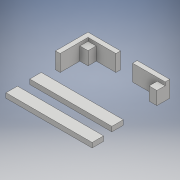
# Autodesk Inventor part: Suporte_proto
Saved by Autodesk Inventor 2018 (Build 220112000, 112)
## iProperties
Created: 2018-05-07
Part Number: Suporte_proto
Material: Genérico
Document SubType Name: Modeling
Designer: mirre
Density: 1 g/cm^3
Appearance: Padrão
Author: mirre
Autodesk Inventor part; units mm, degrees
ref_plane "YZ Plane" through (0, 0, 0) normal (1, 0, 0) x (0, 1, 0)
ref_plane "XZ Plane" through (0, 0, 0) normal (0, 1, 0) x (-1, 0, 0)
ref_plane "XY Plane" through (0, 0, 0) normal (0, 0, 1) x (1, 0, 0)
sketch "Esboço1" plane through (0, 0, 0) normal (0, 0, 1) x (1, 0, 0)
  line L0 (0, 20) -> (0, 0)
  line L1 (45, 0) -> (45, 5)
  line L2 (45, 5) -> (50, 5)
  line L3 (50, 5) -> (50, 0)
  line L4 (50, 0) -> (45, 0)
  line L5 (0, 30) -> (0, 50)
  line L6 (8, 47) -> (8, 42)
  line L7 (8, 42) -> (3, 42)
  line L8 (3, 42) -> (3, 30)
  line L9 (3, 30) -> (0, 30)
  line L10 (30, 50) -> (50, 50)
  line L11 (50, 50) -> (50, 42)
  line L12 (50, 42) -> (45, 42)
  line L13 (45, 42) -> (45, 47)
  line L14 (45, 47) -> (30, 47)
  line L15 (30, 47) -> (30, 50)
  line L16 (0, 50) -> (20, 50)
  line L17 (20, 50) -> (20, 47)
  line L18 (20, 47) -> (8, 47)
  line L19 (0, 20) -> (3, 20)
  line L20 (3, 20) -> (3, 5)
  line L21 (0, 0) -> (8, 0)
  line L22 (8, 0) -> (8, 5)
  line L23 (8, 5) -> (3, 5)
  line L24 (0.1, 49.9) -> (0.1, 30.1)
  line L25 (0.1, 30.1) -> (2.9, 30.1)
  line L26 (2.9, 30.1) -> (2.9, 42.1)
  line L27 (2.9, 42.1) -> (7.9, 42.1)
  line L28 (7.9, 42.1) -> (7.9, 47.1)
  line L29 (7.9, 47.1) -> (19.9, 47.1)
  line L30 (19.9, 47.1) -> (19.9, 49.9)
  line L31 (19.9, 49.9) -> (0.1, 49.9)
  line L32 (30.1, 49.9) -> (30.1, 47.1)
  line L33 (30.1, 47.1) -> (45.1, 47.1)
  line L34 (45.1, 47.1) -> (45.1, 42.1)
  line L35 (45.1, 42.1) -> (49.9, 42.1)
  line L36 (49.9, 42.1) -> (49.9, 49.9)
  line L37 (49.9, 49.9) -> (30.1, 49.9)
  line L38 (45.1, 4.9) -> (45.1, 0.1)
  line L39 (45.1, 0.1) -> (49.9, 0.1)
  line L40 (49.9, 0.1) -> (49.9, 4.9)
  line L41 (49.9, 4.9) -> (45.1, 4.9)
  line L42 (0.1, 19.9) -> (0.1, 0.1)
  line L43 (0.1, 0.1) -> (7.9, 0.1)
  line L44 (7.9, 0.1) -> (7.9, 4.9)
  line L45 (7.9, 4.9) -> (2.9, 4.9)
  line L46 (2.9, 4.9) -> (2.9, 19.9)
  line L47 (2.9, 19.9) -> (0.1, 19.9)
  dimension "d3" = 10
  dimension "d4" = 20
  dimension "d6" = 20
  dimension "d7" = 5
  dimension "d8" = 5
  dimension "d9" = 3
  dimension "d10" = 3
  dimension "d11" = 20
  dimension "d14" = 5
  dimension "d15" = 5
  dimension "d16" = 3
  dimension "d17" = 5
  dimension "d18" = 5
  dimension "d19" = 3
  dimension "d20" = 5
  dimension "d21" = 20
  dimension "d22" = 10
  dimension "d23" = 5
  dimension "d33" = 0.1
  dimension "d34" = 0.1
  dimension "d35" = 0.1
  dimension "d36" = 0.1
  dimension "d37" = 0.1
  dimension "d38" = 0.1
  dimension "d40" = 0.1
  dimension "d41" = 0.1
  dimension "d43" = 0.1
  dimension "d44" = 0.1
  dimension "d45" = 0.1
  dimension "d46" = 0.1
  dimension "d47" = 0.1
  dimension "d48" = 0.1
  dimension "d49" = 0.1
  dimension "d50" = 0.1
  dimension "d51" = 0.1
  dimension "d52" = 0.1
  dimension "d53" = 0.1
  dimension "d54" = 0.1
  dimension "d55" = 0.1
  dimension "d56" = 0.1
  constraints: 96 end point, 32 perpendicular, 8 point on line, 4 parallel, 3 collinear, 3 horizontal, 2 vertical
  measures "d3" distance between parallel lines of L15 L17
  measures "d4" distance from line of L16.end L5
  measures "d6" distance between parallel lines of L16 L9
  measures "d7" distance between parallel lines of L6 L8
  measures "d8" distance between parallel lines of L18 L7
  measures "d9" distance between parallel lines of L16 L18
  measures "d10" distance between parallel lines of L8 L5
  measures "d11" distance between parallel lines of L11 L15
  measures "d14" distance between parallel lines of L12 L14
  measures "d15" distance between parallel lines of L11 L13
  measures "d16" distance between parallel lines of L10 L14
  measures "d17" distance between parallel lines of L3 L1
  measures "d18" distance between parallel lines of L2 L4
  measures "d19" distance of L0.start L19.end
  measures "d20" distance from line of L22.end L20
  measures "d21" distance between parallel lines of L21 L19
  measures "d22" distance between parallel lines of L9 L19
  measures "d23" distance between parallel lines of L23 L21
  measures "d33" distance between parallel lines of L16 L31
  measures "d34" distance between parallel lines of L17 L30
  measures "d35" distance between parallel lines of L18 L29
  measures "d36" distance between parallel lines of L6 L28
  measures "d37" distance between parallel lines of L7 L27
  measures "d38" distance between parallel lines of L8 L26
  measures "d40" distance between parallel lines of L5 L24
  measures "d41" distance between parallel lines of L25 L9
  measures "d43" distance between parallel lines of L10 L37
  measures "d44" distance between parallel lines of L11 L36
  measures "d45" distance between parallel lines of L12 L35
  measures "d46" distance between parallel lines of L13 L34
  measures "d47" distance between parallel lines of L33 L14
  measures "d48" distance between parallel lines of L15 L32
  measures "d49" distance between parallel lines of L1 L38
  measures "d50" distance between parallel lines of L2 L41
  measures "d51" distance between parallel lines of L3 L40
  measures "d52" distance between parallel lines of L4 L39
  measures "d53" distance between parallel lines of L0 L42
  measures "d54" distance between parallel lines of L22 L44
  measures "d55" distance between parallel lines of L20 L46
  measures "d56" distance between parallel lines of L19 L47
extrude "Extrusão3" add sketch "Esboço1" along normal blind 10 contours L31 L30 L29 L28 L27 L26 L25 L24 | L37 L36 L35 L34 L33 L32 | L41 L40 L39 L38 | L47 L46 L45 L44 L43 L42
sketch "Esboço3" plane through (0, 0, 10) normal (0, 0, 1) x (1, 0, 0)
  line L0 (7.9, 0.1) -> (7.9, 4.9) projected
  line L1 (7.9, 4.9) -> (2.9, 4.9)
  line L2 (2.9, 4.9) -> (2.9, 0.1)
  line L3 (2.9, 0.1) -> (7.9, 0.1)
  line L4 (7.9, 0.1) -> (7.9, 4.9)
  line L5 (49.9, 4.9) -> (45.1, 4.9) projected
  line L6 (45.1, 0.1) -> (49.9, 0.1) projected
  line L7 (45.1, 4.9) -> (49.9, 4.9)
  line L8 (49.9, 4.9) -> (49.9, 0.1)
  line L9 (49.9, 0.1) -> (45.1, 0.1)
  line L10 (45.1, 0.1) -> (45.1, 4.9)
  line L11 (50.9, 47.1) -> (45.1, 47.1)
  line L12 (46.1, 42.1) -> (49.9, 42.1)
  line L13 (45.1, 47.1) -> (49.9, 47.1)
  line L14 (49.9, 47.1) -> (49.9, 42.1)
  line L15 (49.9, 42.1) -> (45.1, 42.1)
  line L16 (45.1, 42.1) -> (45.1, 47.1)
  line L17 (45.1, 42.1) -> (49.9, 42.1) projected
  line L18 (49.9, 42.1) -> (49.9, 49.9) projected
  line L19 (7.9, 42.1) -> (2.9, 42.1)
  line L20 (2.9, 42.1) -> (2.9, 47.1)
  line L21 (2.9, 47.1) -> (7.9, 47.1)
  line L22 (7.9, 47.1) -> (7.9, 42.1)
  line L23 (7.9, 47.1) -> (19.9, 47.1) projected
  line L24 (2.9, 30.1) -> (2.9, 42.1) projected
  point P0 (0, 0)
  dimension "d60" = 4.8
  dimension "d61" = 5
  dimension "d62" = 4.8
  dimension "d63" = 5
  constraints: 36 end point, 8 parallel, 4 collinear, 4 horizontal, 4 perpendicular
  measures "d60" distance between parallel lines of L1 L3
  measures "d61" distance between parallel lines of L11 L12
  measures "d62" distance between parallel lines of L16 L14
  measures "d63" distance between parallel lines of L0 L2
extrude "Extrusão4" cut sketch "Esboço3" against normal blind 2
sketch "Esboço4" plane through (0, 0, 10) normal (0, 0, 1) x (1, 0, 0)
  line L0 (-10.899, 26.671) -> (68.9569, 26.671)
  line L1 (68.9569, 26.671) -> (68.9569, -16.1913)
  line L2 (68.9569, -16.1913) -> (-10.899, -16.1913)
  line L3 (-10.899, -16.1913) -> (-10.899, 26.671)
  point P0 (0, 0)
  constraints: 8 end point, 2 parallel, 1 horizontal, 1 perpendicular
extrude "Extrusão5" cut sketch "Esboço4" against normal blind 20
sketch "Esboço5" plane through (0, 0, 0) normal (0, 0, -1) x (-1, 0, 0)
  line L0 (0, 0) -> (-52.5, 0)
  line L1 (-52.5, 0) -> (-52.5, 7)
  line L2 (-52.5, 7) -> (0, 7)
  line L3 (0, 7) -> (0, 0)
  line L4 (0, 21.5) -> (-50, 21.5)
  line L5 (-50, 21.5) -> (-50, 14.5)
  line L6 (-50, 14.5) -> (0, 14.5)
  line L7 (0, 14.5) -> (0, 21.5)
  line L8 (-0.1, 30.1) -> (-2.9, 30.1) projected
  dimension "d68" = 52.5
  dimension "d69" = 50
  dimension "d72" = 7
  dimension "d73" = 7
  dimension "d74" = 7.5
  constraints: 16 end point, 4 parallel, 2 horizontal, 2 perpendicular, 1 collinear
  measures "d68" distance between parallel lines of L1 L3
  measures "d69" distance between parallel lines of L5 L7
  measures "d72" distance between parallel lines of L6 L4
  measures "d73" distance between parallel lines of L2 L0
  measures "d74" distance between parallel lines of L6 L2
extrude "Extrusão6" add sketch "Esboço5" against normal blind 2.9
